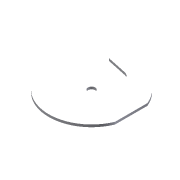
# Autodesk Inventor part: OpenROV 2_3_2 Dev EndCap 108
Saved by Autodesk Inventor 2012 (Build 160160000, 160)
## iProperties
Created: 2011-09-29
Part Number: OpenROV 2_3_2 Dev EndCap 108
Document SubType Name: Modeling
Designer: user
Density: 1 g/cm^3
Material: Default
Author: user
Autodesk Inventor part; units mm, degrees
ref_plane "YZ Plane" through (0, 0, 0) normal (1, 0, 0) x (0, 1, 0)
ref_plane "XZ Plane" through (0, 0, 0) normal (0, 1, 0) x (-1, 0, 0)
ref_plane "XY Plane" through (0, 0, 0) normal (0, 0, 1) x (1, 0, 0)
sketch "Sketch1" plane through (0, 0, 0) normal (0, 0, 1) x (1, 0, 0)
  circle A0 centre (0, 0) radius 4.59
  arc A1 (-2.0962, 20.2222) -> (2.0962, 39.7778) centre (0, 30) ccw
  line L0 (2.0962, 39.7778) -> (-22.6062, 45.0736)
  line L1 (-2.0962, 20.2222) -> (-43.8842, 29.1807)
  line L2 (50, -20) -> (50, 20)
  arc A2 (-46.0074, 28.2723) -> (49.8462, -20.7692) centre (0, 0) ccw
  arc A3 (49.8462, 20.7692) -> (-23.0403, 48.8379) centre (0, 0) ccw
  arc A4 (-43.8842, 29.1807) -> (-46.0074, 28.2723) centre (-44.3034, 27.2252) ccw
  arc A5 (-23.0403, 48.8379) -> (-22.6062, 45.0736) centre (-22.187, 47.0291) ccw
  arc A6 (50, 20) -> (49.8462, 20.7692) centre (48, 20) ccw
  arc A7 (49.8462, -20.7692) -> (50, -20) centre (48, -20) ccw
  point P0 (-27.9313, 46.2152)
  point P1 (-45.2476, 29.473)
  point P2 (50, -20.3961)
  point P3 (50, 20.3961)
  dimension "d1" = 9.18
  dimension "d4" = 20
  dimension "d5" = 30
  dimension "d12" = 50
  dimension "d13" = 2
  dimension "d14" = 54
  dimension "d15" = 54
  dimension "d16" = 20
  dimension "d19" = 77.9
  dimension "d20" = 50
  constraints: 19 point on circle, 9 tangent, 8 centre point, 6 end point, 5 point on line, 3 equal radius, 2 coincident, 1 parallel, 1 vertical
  measures "d1" diameter of A0
  measures "d4" diameter of A1
  measures "d5" distance of A0.centre A1.centre
  measures "d12" distance from line of point (0, 0) L2
  measures "d13" radius of A4
  measures "d14" radius of A2
  measures "d15" radius of A3
  measures "d16" distance between parallel lines of L0 L1
  measures "d19" angle of L0 L2
  measures "d20" distance from line of A1.centre L2
extrude "Extrusion3" add sketch "Sketch1" along normal blind 3
body "Solid3"
